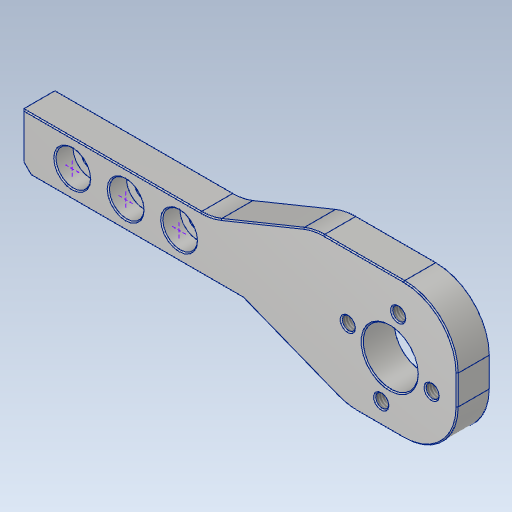
# Autodesk Inventor part: Xmovementarm
Saved by Autodesk Inventor 2020 (Build 240168000, 168)
## iProperties
Created: 2019-01-13
Part Number: Xmovementarm
Material: Aluminum 6061
Document SubType Name: Modeling
Designer: LillaHunden
Density: 2.7 g/cm^3
Appearance: Aluminum - Flat
Mass: 17.0465 g
Surface Area: 40.0048 cm^2
Volume: 6.31351 cm^3
Author: LillaHunden
Autodesk Inventor part; units mm, degrees
ref_plane "YZ Plane" through (0, 0, 0) normal (1, 0, 0) x (0, 1, 0)
ref_plane "XZ Plane" through (0, 0, 0) normal (0, 1, 0) x (-1, 0, 0)
ref_plane "XY Plane" through (0, 0, 0) normal (0, 0, 1) x (1, 0, 0)
sketch "Sketch1" plane through (0, 0, 0) normal (0, 0, 1) x (1, 0, 0)
  line L0 (86.0355, 17.7845) -> (59.096, 17.7845)
  line L1 (59.096, 17.7845) -> (59.096, 0)
  line L2 (65.4983, -7.6947) -> (86.0355, -7.6947)
  line L3 (86.0355, -7.6947) -> (86.0355, 17.7845)
  line L4 (6.25, 0) -> (40, 0) projected
  line L5 (40, 0) -> (40, 10) projected
  line L6 (4.75, 10) -> (40, 10) projected
  line L7 (40, 10) -> (59.096, 10)
  line L8 (40, 0) -> (59.096, 0)
  line L9 (59.096, 17.7845) -> (40, 10)
  circle A0 centre (34, 5) radius 2 projected
  line L10 (4.75, 10) -> (4.75, 1.5) projected
  circle A1 centre (14, 5) radius 1.5 projected
  circle A2 centre (34, 5) radius 1.5 projected
  circle A3 centre (24, 5) radius 1.5 projected
  line L11 (6.25, 0) -> (4.75, 1.5) projected
  line L12 (46, -2.9015) -> (46, 0) projected
  line L13 (65.4983, -7.6947) -> (46, 0)
  constraints: 16 end point, 3 perpendicular, 2 parallel, 1 horizontal, 1 point on line, 1 vertical alignment
extrude "Extrusion1" add sketch "Sketch1" along normal blind 6 contours L3 L2 L13 L8 L1 L0 | L1 L7 L9 | L1 L8 L5 L7 | L5 L4 L11 L10 L6 | A0 | A1 | A2 | A3
sketch "Sketch2" plane through (0, 0, 0) normal (0, 0, -1) x (-1, 0, 0)
  circle A0 centre (-73.4131, 4.0423) radius 11 construction
  spline S0 degree 3 poles (-70.2966, -4.0075) (-70.3394, -4.1944) (-70.4189, -4.3706) (-70.5284, -4.5282) (-70.5355, -4.5385) (-70.5428, -4.5487) (-70.5503, -4.5589) (-70.6442, -4.6873) (-70.7571, -4.8004) (-70.8853, -4.8928) (-70.903, -4.9055) (-70.921, -4.9179) (-70.9392, -4.9298) (-70.9477, -4.9354) (-70.9563, -4.9408) (-70.9649, -4.9462) (-71.0438, -4.9954) (-71.1272, -5.0364) (-71.2142, -5.0682) (-71.2658, -5.087) (-71.3187, -5.1025) (-71.3725, -5.1148) (-71.4037, -5.1219) (-71.4353, -5.1279) (-71.4671, -5.1328) (-71.6122, -5.1551) (-71.7606, -5.1543) (-71.906, -5.1306) (-71.9241, -5.1277) (-71.9422, -5.1244) (-71.9602, -5.1207) (-71.9711, -5.1185) (-71.9819, -5.1162) (-71.9928, -5.1137) (-72.0898, -5.0915) (-72.1841, -5.059) (-72.2734, -5.016) (-72.3457, -4.9813) (-72.4143, -4.9399) (-72.478, -4.8918) (-72.4941, -4.8797) (-72.5098, -4.8672) (-72.5244, -4.8525) knots 0 0 0 0 0.200829 0.200829 0.200829 0.213978 0.213978 0.213978 0.380655 0.380655 0.380655 0.403633 0.403633 0.403633 0.414319 0.414319 0.414319 0.512539 0.512539 0.512539 0.570815 0.570815 0.570815 0.60461 0.60461 0.60461 0.759068 0.759068 0.759068 0.77833 0.77833 0.77833 0.789949 0.789949 0.789949 0.894318 0.894318 0.894318 0.978751 0.978751 0.978751 1 1 1 1 construction
  arc A1 (-73.0648, -4.0495) -> (-72.5243, -4.8523) centre (-71.8254, -3.7985) ccw construction
  spline S1 degree 3 poles (-73.0648, -4.0495) (-73.1089, -3.9109) (-73.127, -3.7658) (-73.1216, -3.6205) (-73.121, -3.6026) (-73.12, -3.5847) (-73.1186, -3.5668) (-73.1178, -3.5567) (-73.117, -3.5466) (-73.116, -3.5366) (-73.1013, -3.3878) (-73.0625, -3.2423) (-73.0016, -3.1063) (-72.9947, -3.091) (-72.9875, -3.0757) (-72.9801, -3.0606) (-72.9752, -3.0506) (-72.9701, -3.0407) (-72.9649, -3.0308) (-72.923, -2.9506) (-72.8732, -2.8752) (-72.8161, -2.8057) (-72.7812, -2.7633) (-72.7435, -2.7231) (-72.7034, -2.6852) (-72.6914, -2.6738) (-72.6792, -2.6627) (-72.6668, -2.6518) (-72.6553, -2.6417) (-72.6436, -2.6318) (-72.6317, -2.622) (-72.5007, -2.5145) (-72.3507, -2.4308) (-72.19, -2.3729) (-72.1789, -2.3689) (-72.1678, -2.365) (-72.1566, -2.3613) (-72.062, -2.3296) (-71.9647, -2.3072) (-71.8662, -2.2944) (-71.8501, -2.2924) (-71.8341, -2.2905) (-71.818, -2.289) (-71.8062, -2.2878) (-71.7944, -2.2868) (-71.7826, -2.286) (-71.722, -2.2815) (-71.6612, -2.2808) (-71.6007, -2.2839) (-71.5723, -2.2854) (-71.544, -2.2877) (-71.5158, -2.2909) (-71.4916, -2.2936) (-71.4675, -2.297) (-71.4437, -2.3035) knots 0 0 0 0 0.153066 0.153066 0.153066 0.171917 0.171917 0.171917 0.182531 0.182531 0.182531 0.339556 0.339556 0.339556 0.35729 0.35729 0.35729 0.369023 0.369023 0.369023 0.464442 0.464442 0.464442 0.522742 0.522742 0.522742 0.540193 0.540193 0.540193 0.556325 0.556325 0.556325 0.734813 0.734813 0.734813 0.747126 0.747126 0.747126 0.851246 0.851246 0.851246 0.868176 0.868176 0.868176 0.880588 0.880588 0.880588 0.944403 0.944403 0.944403 0.974326 0.974326 0.974326 1 1 1 1 construction
  arc A2 (-70.2966, -4.0075) -> (-71.4439, -2.3035) centre (-71.8254, -3.7985) ccw construction
  spline S2 degree 3 poles (-64.0434, 5.421) (-64.0862, 5.2342) (-64.1657, 5.0579) (-64.2751, 4.9003) (-64.2823, 4.89) (-64.2896, 4.8798) (-64.297, 4.8697) (-64.404, 4.7235) (-64.5353, 4.5971) (-64.686, 4.4987) (-64.6945, 4.4932) (-64.703, 4.4877) (-64.7116, 4.4824) (-64.7906, 4.4331) (-64.874, 4.3921) (-64.9609, 4.3604) (-65.0125, 4.3415) (-65.0654, 4.326) (-65.1193, 4.3137) (-65.1359, 4.31) (-65.1526, 4.3065) (-65.1694, 4.3033) (-65.1842, 4.3006) (-65.199, 4.298) (-65.2138, 4.2957) (-65.359, 4.2734) (-65.5074, 4.2742) (-65.6528, 4.2979) (-65.6709, 4.3008) (-65.689, 4.3041) (-65.707, 4.3078) (-65.7179, 4.31) (-65.7287, 4.3124) (-65.7395, 4.3148) (-65.8246, 4.3343) (-65.9075, 4.3617) (-65.9869, 4.3971) (-65.9981, 4.402) (-66.0092, 4.4072) (-66.0202, 4.4125) (-66.0665, 4.4348) (-66.1114, 4.4598) (-66.1544, 4.4876) (-66.1784, 4.5031) (-66.2019, 4.5195) (-66.2248, 4.5367) (-66.2409, 4.5488) (-66.2566, 4.5613) (-66.2712, 4.576) knots 0 0 0 0 0.200829 0.200829 0.200829 0.213978 0.213978 0.213978 0.403633 0.403633 0.403633 0.414319 0.414319 0.414319 0.512539 0.512539 0.512539 0.570815 0.570815 0.570815 0.588808 0.588808 0.588808 0.60461 0.60461 0.60461 0.759068 0.759068 0.759068 0.77833 0.77833 0.77833 0.789949 0.789949 0.789949 0.881423 0.881423 0.881423 0.894318 0.894318 0.894318 0.948472 0.948472 0.948472 0.978751 0.978751 0.978751 1 1 1 1 construction
  arc A3 (-66.8115, 5.379) -> (-66.2711, 4.5762) centre (-65.5722, 5.63) ccw construction
  spline S3 degree 3 poles (-66.8115, 5.379) (-66.8557, 5.5177) (-66.8737, 5.6627) (-66.8684, 5.808) (-66.8678, 5.8259) (-66.8667, 5.8438) (-66.8654, 5.8617) (-66.8646, 5.8718) (-66.8637, 5.8819) (-66.8627, 5.892) (-66.848, 6.0407) (-66.8092, 6.1862) (-66.7483, 6.3222) (-66.7415, 6.3376) (-66.7343, 6.3528) (-66.7269, 6.3679) (-66.7219, 6.3779) (-66.7169, 6.3879) (-66.7117, 6.3977) (-66.6697, 6.4779) (-66.62, 6.5534) (-66.5629, 6.6228) (-66.528, 6.6653) (-66.4903, 6.7055) (-66.4502, 6.7433) (-66.4382, 6.7547) (-66.426, 6.7658) (-66.4135, 6.7767) (-66.402, 6.7868) (-66.3903, 6.7968) (-66.3785, 6.8065) (-66.2625, 6.9017) (-66.1315, 6.9782) (-65.9915, 7.0347) (-65.9734, 7.042) (-65.9552, 7.049) (-65.9368, 7.0556) (-65.8689, 7.0801) (-65.7992, 7.0998) (-65.7287, 7.1145) (-65.6904, 7.1225) (-65.6518, 7.1291) (-65.6129, 7.1341) (-65.5969, 7.1362) (-65.5809, 7.138) (-65.5648, 7.1396) (-65.553, 7.1407) (-65.5412, 7.1417) (-65.5294, 7.1426) (-65.4687, 7.147) (-65.408, 7.1477) (-65.3475, 7.1446) (-65.3191, 7.1431) (-65.2908, 7.1408) (-65.2626, 7.1376) (-65.2384, 7.1349) (-65.2142, 7.1316) (-65.1905, 7.125) knots 0 0 0 0 0.153066 0.153066 0.153066 0.171917 0.171917 0.171917 0.182531 0.182531 0.182531 0.339556 0.339556 0.339556 0.35729 0.35729 0.35729 0.369023 0.369023 0.369023 0.464442 0.464442 0.464442 0.522742 0.522742 0.522742 0.540193 0.540193 0.540193 0.556325 0.556325 0.556325 0.714368 0.714368 0.714368 0.734813 0.734813 0.734813 0.810219 0.810219 0.810219 0.851246 0.851246 0.851246 0.868176 0.868176 0.868176 0.880588 0.880588 0.880588 0.944403 0.944403 0.944403 0.974325 0.974325 0.974325 1 1 1 1 construction
  arc A4 (-64.0434, 5.421) -> (-65.1906, 7.1251) centre (-65.5722, 5.63) ccw construction
  spline S4 degree 3 poles (-73.4719, 11.6743) (-73.5094, 11.5106) (-73.5751, 11.3552) (-73.6643, 11.2132) (-73.6769, 11.193) (-73.6901, 11.1732) (-73.7037, 11.1536) (-73.7108, 11.1433) (-73.7181, 11.133) (-73.7255, 11.1229) (-73.8195, 10.9944) (-73.9324, 10.8814) (-74.0606, 10.789) (-74.0783, 10.7762) (-74.0963, 10.7639) (-74.1145, 10.752) (-74.123, 10.7464) (-74.1315, 10.741) (-74.1401, 10.7356) (-74.2191, 10.6864) (-74.3025, 10.6453) (-74.3895, 10.6136) (-74.4411, 10.5948) (-74.4939, 10.5792) (-74.5478, 10.567) (-74.5644, 10.5632) (-74.5811, 10.5597) (-74.5979, 10.5566) (-74.7569, 10.5267) (-74.921, 10.5251) (-75.0813, 10.5511) (-75.0994, 10.5541) (-75.1175, 10.5574) (-75.1355, 10.561) (-75.1464, 10.5633) (-75.1572, 10.5656) (-75.168, 10.5681) (-75.2531, 10.5875) (-75.3361, 10.6149) (-75.4154, 10.6503) (-75.4266, 10.6553) (-75.4377, 10.6604) (-75.4487, 10.6657) (-75.521, 10.7005) (-75.5896, 10.7418) (-75.6533, 10.7899) (-75.6694, 10.802) (-75.6851, 10.8146) (-75.6997, 10.8292) knots 0 0 0 0 0.175859 0.175859 0.175859 0.200829 0.200829 0.200829 0.213978 0.213978 0.213978 0.380655 0.380655 0.380655 0.403633 0.403633 0.403633 0.414319 0.414319 0.414319 0.512539 0.512539 0.512539 0.570815 0.570815 0.570815 0.588808 0.588808 0.588808 0.759068 0.759068 0.759068 0.77833 0.77833 0.77833 0.789949 0.789949 0.789949 0.881423 0.881423 0.881423 0.894318 0.894318 0.894318 0.978751 0.978751 0.978751 1 1 1 1 construction
  arc A5 (-76.2401, 11.6323) -> (-75.6996, 10.8294) centre (-75.0007, 11.8832) ccw construction
  spline S5 degree 3 poles (-76.2401, 11.6323) (-76.2927, 11.7976) (-76.3084, 11.9722) (-76.2913, 12.1452) (-76.2765, 12.294) (-76.2378, 12.4394) (-76.1769, 12.5754) (-76.17, 12.5908) (-76.1628, 12.606) (-76.1554, 12.6212) (-76.1505, 12.6312) (-76.1454, 12.6411) (-76.1402, 12.6509) (-76.0982, 12.7311) (-76.0485, 12.8066) (-75.9914, 12.8761) (-75.9565, 12.9185) (-75.9188, 12.9587) (-75.8787, 12.9966) (-75.8667, 13.0079) (-75.8545, 13.019) (-75.842, 13.03) (-75.8305, 13.0401) (-75.8189, 13.05) (-75.807, 13.0597) (-75.691, 13.155) (-75.5601, 13.2315) (-75.4201, 13.288) (-75.402, 13.2953) (-75.3837, 13.3022) (-75.3653, 13.3089) (-75.3542, 13.3129) (-75.3431, 13.3167) (-75.3319, 13.3205) (-75.2373, 13.3521) (-75.14, 13.3746) (-75.0415, 13.3873) (-75.0254, 13.3894) (-75.0094, 13.3912) (-74.9933, 13.3928) (-74.9815, 13.3939) (-74.9697, 13.3949) (-74.9579, 13.3958) (-74.8688, 13.4023) (-74.7795, 13.4008) (-74.6911, 13.3909) (-74.6669, 13.3882) (-74.6427, 13.3848) (-74.619, 13.3783) knots 0 0 0 0 0.182531 0.182531 0.182531 0.339556 0.339556 0.339556 0.357289 0.357289 0.357289 0.369023 0.369023 0.369023 0.464442 0.464442 0.464442 0.522742 0.522742 0.522742 0.540193 0.540193 0.540193 0.556325 0.556325 0.556325 0.714368 0.714368 0.714368 0.734813 0.734813 0.734813 0.747125 0.747125 0.747125 0.851246 0.851246 0.851246 0.868176 0.868176 0.868176 0.880588 0.880588 0.880588 0.974325 0.974325 0.974325 1 1 1 1 construction
  arc A6 (-73.4719, 11.6743) -> (-74.6192, 13.3783) centre (-75.0007, 11.8832) ccw construction
  spline S6 degree 3 poles (-79.7252, 2.2457) (-79.8062, 1.8916) (-80.0211, 1.5714) (-80.3139, 1.3604) (-80.3315, 1.3477) (-80.3495, 1.3354) (-80.3677, 1.3234) (-80.3762, 1.3179) (-80.3848, 1.3124) (-80.3934, 1.3071) (-80.4724, 1.2579) (-80.5557, 1.2168) (-80.6427, 1.1851) (-80.6943, 1.1662) (-80.7472, 1.1507) (-80.801, 1.1385) (-80.8177, 1.1347) (-80.8344, 1.1312) (-80.8512, 1.128) (-80.8659, 1.1253) (-80.8807, 1.1227) (-80.8956, 1.1204) (-81.0408, 1.0981) (-81.1891, 1.0989) (-81.3345, 1.1226) (-81.3526, 1.1256) (-81.3707, 1.1289) (-81.3888, 1.1325) (-81.3996, 1.1347) (-81.4105, 1.1371) (-81.4213, 1.1395) (-81.5064, 1.159) (-81.5893, 1.1864) (-81.6686, 1.2218) (-81.6798, 1.2268) (-81.6909, 1.2319) (-81.702, 1.2372) (-81.7742, 1.2719) (-81.8428, 1.3133) (-81.9066, 1.3614) (-81.9226, 1.3735) (-81.9384, 1.3861) (-81.953, 1.4007) knots 0 0 0 0 0.380655 0.380655 0.380655 0.403633 0.403633 0.403633 0.414319 0.414319 0.414319 0.512539 0.512539 0.512539 0.570815 0.570815 0.570815 0.588808 0.588808 0.588808 0.60461 0.60461 0.60461 0.759068 0.759068 0.759068 0.77833 0.77833 0.77833 0.789949 0.789949 0.789949 0.881423 0.881423 0.881423 0.894318 0.894318 0.894318 0.978751 0.978751 0.978751 1 1 1 1 construction
  arc A7 (-82.4933, 2.2038) -> (-81.9529, 1.4009) centre (-81.2539, 2.4547) ccw construction
  spline S7 degree 3 poles (-82.4933, 2.2038) (-82.5374, 2.3424) (-82.5555, 2.4874) (-82.5502, 2.6328) (-82.5495, 2.6507) (-82.5485, 2.6686) (-82.5471, 2.6865) (-82.5464, 2.6965) (-82.5455, 2.7066) (-82.5445, 2.7167) (-82.5281, 2.8823) (-82.482, 3.0437) (-82.4086, 3.1926) (-82.4037, 3.2026) (-82.3986, 3.2126) (-82.3935, 3.2224) (-82.3515, 3.3026) (-82.3017, 3.3781) (-82.2446, 3.4475) (-82.2097, 3.49) (-82.1721, 3.5302) (-82.132, 3.5681) (-82.1199, 3.5794) (-82.1077, 3.5905) (-82.0953, 3.6014) (-82.0838, 3.6115) (-82.0721, 3.6215) (-82.0603, 3.6312) (-81.9292, 3.7388) (-81.7792, 3.8225) (-81.6185, 3.8803) (-81.6074, 3.8843) (-81.5963, 3.8882) (-81.5851, 3.892) (-81.4752, 3.9287) (-81.3615, 3.9531) (-81.2465, 3.9643) (-81.2348, 3.9654) (-81.223, 3.9664) (-81.2111, 3.9673) (-81.1505, 3.9717) (-81.0897, 3.9724) (-81.0292, 3.9693) (-81.0009, 3.9678) (-80.9726, 3.9655) (-80.9443, 3.9624) (-80.9201, 3.9596) (-80.896, 3.9563) (-80.8722, 3.9497) knots 0 0 0 0 0.153066 0.153066 0.153066 0.171917 0.171917 0.171917 0.182531 0.182531 0.182531 0.357289 0.357289 0.357289 0.369023 0.369023 0.369023 0.464442 0.464442 0.464442 0.522742 0.522742 0.522742 0.540193 0.540193 0.540193 0.556325 0.556325 0.556325 0.734813 0.734813 0.734813 0.747125 0.747125 0.747125 0.868176 0.868176 0.868176 0.880588 0.880588 0.880588 0.944403 0.944403 0.944403 0.974325 0.974325 0.974325 1 1 1 1 construction
  arc A8 (-79.7252, 2.2457) -> (-80.8724, 3.9498) centre (-81.2539, 2.4547) ccw construction
  circle A9 centre (-73.4131, 4.0423) radius 5.15 construction
  point P0 (0, 0)
  constraints: 4 coincident
hole "Hole1" at (81.2539, 2.4547, 0) at (75.0007, 11.8832, 0) at (65.5722, 5.63, 0) at (71.8254, -3.7985, 0) direction (0, 0, 1) diameter 2.459 depth 8.8 thread size "M3x0.5" class "6H" standard "ISO Metric profile"
sketch "Sketch3" plane through (0, 0, 6) normal (0, 0, 1) x (1, 0, 0)
  circle A0 centre (73.4131, 4.0423) radius 11
  spline S0 degree 3 poles (70.2966, -4.0075) (70.3394, -4.1944) (70.4189, -4.3706) (70.5284, -4.5282) (70.5355, -4.5385) (70.5428, -4.5487) (70.5503, -4.5589) (70.6442, -4.6873) (70.7571, -4.8004) (70.8853, -4.8928) (70.903, -4.9055) (70.921, -4.9179) (70.9392, -4.9298) (70.9477, -4.9354) (70.9563, -4.9408) (70.9649, -4.9462) (71.0438, -4.9954) (71.1272, -5.0364) (71.2142, -5.0682) (71.2658, -5.087) (71.3187, -5.1025) (71.3725, -5.1148) (71.4037, -5.1219) (71.4353, -5.1279) (71.4671, -5.1328) (71.6122, -5.1551) (71.7606, -5.1543) (71.906, -5.1306) (71.9241, -5.1277) (71.9422, -5.1244) (71.9602, -5.1207) (71.9711, -5.1185) (71.9819, -5.1162) (71.9928, -5.1137) (72.0898, -5.0915) (72.1841, -5.059) (72.2734, -5.016) (72.3457, -4.9813) (72.4143, -4.9399) (72.478, -4.8918) (72.4941, -4.8797) (72.5098, -4.8672) (72.5244, -4.8525) knots 0 0 0 0 0.200829 0.200829 0.200829 0.213978 0.213978 0.213978 0.380655 0.380655 0.380655 0.403633 0.403633 0.403633 0.414319 0.414319 0.414319 0.512539 0.512539 0.512539 0.570815 0.570815 0.570815 0.60461 0.60461 0.60461 0.759068 0.759068 0.759068 0.77833 0.77833 0.77833 0.789949 0.789949 0.789949 0.894318 0.894318 0.894318 0.978751 0.978751 0.978751 1 1 1 1
  arc A1 (72.5243, -4.8523) -> (73.0648, -4.0495) centre (71.8254, -3.7985) ccw
  spline S1 degree 3 poles (73.0648, -4.0495) (73.1089, -3.9109) (73.127, -3.7658) (73.1216, -3.6205) (73.121, -3.6026) (73.12, -3.5847) (73.1186, -3.5668) (73.1178, -3.5567) (73.117, -3.5466) (73.116, -3.5366) (73.1013, -3.3878) (73.0625, -3.2423) (73.0016, -3.1063) (72.9947, -3.091) (72.9875, -3.0757) (72.9801, -3.0606) (72.9752, -3.0506) (72.9701, -3.0407) (72.9649, -3.0308) (72.923, -2.9506) (72.8732, -2.8752) (72.8161, -2.8057) (72.7812, -2.7633) (72.7435, -2.7231) (72.7034, -2.6852) (72.6914, -2.6738) (72.6792, -2.6627) (72.6668, -2.6518) (72.6553, -2.6417) (72.6436, -2.6318) (72.6317, -2.622) (72.5007, -2.5145) (72.3507, -2.4308) (72.19, -2.3729) (72.1789, -2.3689) (72.1678, -2.365) (72.1566, -2.3613) (72.062, -2.3296) (71.9647, -2.3072) (71.8662, -2.2944) (71.8501, -2.2924) (71.8341, -2.2905) (71.818, -2.289) (71.8062, -2.2878) (71.7944, -2.2868) (71.7826, -2.286) (71.722, -2.2815) (71.6612, -2.2808) (71.6007, -2.2839) (71.5723, -2.2854) (71.544, -2.2877) (71.5158, -2.2909) (71.4916, -2.2936) (71.4675, -2.297) (71.4437, -2.3035) knots 0 0 0 0 0.153066 0.153066 0.153066 0.171917 0.171917 0.171917 0.182531 0.182531 0.182531 0.339556 0.339556 0.339556 0.35729 0.35729 0.35729 0.369023 0.369023 0.369023 0.464442 0.464442 0.464442 0.522742 0.522742 0.522742 0.540193 0.540193 0.540193 0.556325 0.556325 0.556325 0.734813 0.734813 0.734813 0.747126 0.747126 0.747126 0.851246 0.851246 0.851246 0.868176 0.868176 0.868176 0.880588 0.880588 0.880588 0.944403 0.944403 0.944403 0.974326 0.974326 0.974326 1 1 1 1
  arc A2 (71.4439, -2.3035) -> (70.2966, -4.0075) centre (71.8254, -3.7985) ccw
  spline S2 degree 3 poles (64.0434, 5.421) (64.0862, 5.2342) (64.1657, 5.0579) (64.2751, 4.9003) (64.2823, 4.89) (64.2896, 4.8798) (64.297, 4.8697) (64.404, 4.7235) (64.5353, 4.5971) (64.686, 4.4987) (64.6945, 4.4932) (64.703, 4.4877) (64.7116, 4.4824) (64.7906, 4.4331) (64.874, 4.3921) (64.9609, 4.3604) (65.0125, 4.3415) (65.0654, 4.326) (65.1193, 4.3137) (65.1359, 4.31) (65.1526, 4.3065) (65.1694, 4.3033) (65.1842, 4.3006) (65.199, 4.298) (65.2138, 4.2957) (65.359, 4.2734) (65.5074, 4.2742) (65.6528, 4.2979) (65.6709, 4.3008) (65.689, 4.3041) (65.707, 4.3078) (65.7179, 4.31) (65.7287, 4.3124) (65.7395, 4.3148) (65.8246, 4.3343) (65.9075, 4.3617) (65.9869, 4.3971) (65.9981, 4.402) (66.0092, 4.4072) (66.0202, 4.4125) (66.0665, 4.4348) (66.1114, 4.4598) (66.1544, 4.4876) (66.1784, 4.5031) (66.2019, 4.5195) (66.2248, 4.5367) (66.2409, 4.5488) (66.2566, 4.5613) (66.2712, 4.576) knots 0 0 0 0 0.200829 0.200829 0.200829 0.213978 0.213978 0.213978 0.403633 0.403633 0.403633 0.414319 0.414319 0.414319 0.512539 0.512539 0.512539 0.570815 0.570815 0.570815 0.588808 0.588808 0.588808 0.60461 0.60461 0.60461 0.759068 0.759068 0.759068 0.77833 0.77833 0.77833 0.789949 0.789949 0.789949 0.881423 0.881423 0.881423 0.894318 0.894318 0.894318 0.948472 0.948472 0.948472 0.978751 0.978751 0.978751 1 1 1 1
  arc A3 (66.2711, 4.5762) -> (66.8115, 5.379) centre (65.5722, 5.63) ccw
  spline S3 degree 3 poles (66.8115, 5.379) (66.8557, 5.5177) (66.8737, 5.6627) (66.8684, 5.808) (66.8678, 5.8259) (66.8667, 5.8438) (66.8654, 5.8617) (66.8646, 5.8718) (66.8637, 5.8819) (66.8627, 5.892) (66.848, 6.0407) (66.8092, 6.1862) (66.7483, 6.3222) (66.7415, 6.3376) (66.7343, 6.3528) (66.7269, 6.3679) (66.7219, 6.3779) (66.7169, 6.3879) (66.7117, 6.3977) (66.6697, 6.4779) (66.62, 6.5534) (66.5629, 6.6228) (66.528, 6.6653) (66.4903, 6.7055) (66.4502, 6.7433) (66.4382, 6.7547) (66.426, 6.7658) (66.4135, 6.7767) (66.402, 6.7868) (66.3903, 6.7968) (66.3785, 6.8065) (66.2625, 6.9017) (66.1315, 6.9782) (65.9915, 7.0347) (65.9734, 7.042) (65.9552, 7.049) (65.9368, 7.0556) (65.8689, 7.0801) (65.7992, 7.0998) (65.7287, 7.1145) (65.6904, 7.1225) (65.6518, 7.1291) (65.6129, 7.1341) (65.5969, 7.1362) (65.5809, 7.138) (65.5648, 7.1396) (65.553, 7.1407) (65.5412, 7.1417) (65.5294, 7.1426) (65.4687, 7.147) (65.408, 7.1477) (65.3475, 7.1446) (65.3191, 7.1431) (65.2908, 7.1408) (65.2626, 7.1376) (65.2384, 7.1349) (65.2142, 7.1316) (65.1905, 7.125) knots 0 0 0 0 0.153066 0.153066 0.153066 0.171917 0.171917 0.171917 0.182531 0.182531 0.182531 0.339556 0.339556 0.339556 0.35729 0.35729 0.35729 0.369023 0.369023 0.369023 0.464442 0.464442 0.464442 0.522742 0.522742 0.522742 0.540193 0.540193 0.540193 0.556325 0.556325 0.556325 0.714368 0.714368 0.714368 0.734813 0.734813 0.734813 0.810219 0.810219 0.810219 0.851246 0.851246 0.851246 0.868176 0.868176 0.868176 0.880588 0.880588 0.880588 0.944403 0.944403 0.944403 0.974325 0.974325 0.974325 1 1 1 1
  arc A4 (65.1906, 7.1251) -> (64.0434, 5.421) centre (65.5722, 5.63) ccw
  spline S4 degree 3 poles (73.4719, 11.6743) (73.5094, 11.5106) (73.5751, 11.3552) (73.6643, 11.2132) (73.6769, 11.193) (73.6901, 11.1732) (73.7037, 11.1536) (73.7108, 11.1433) (73.7181, 11.133) (73.7255, 11.1229) (73.8195, 10.9944) (73.9324, 10.8814) (74.0606, 10.789) (74.0783, 10.7762) (74.0963, 10.7639) (74.1145, 10.752) (74.123, 10.7464) (74.1315, 10.741) (74.1401, 10.7356) (74.2191, 10.6864) (74.3025, 10.6453) (74.3895, 10.6136) (74.4411, 10.5948) (74.4939, 10.5792) (74.5478, 10.567) (74.5644, 10.5632) (74.5811, 10.5597) (74.5979, 10.5566) (74.7569, 10.5267) (74.921, 10.5251) (75.0813, 10.5511) (75.0994, 10.5541) (75.1175, 10.5574) (75.1355, 10.561) (75.1464, 10.5633) (75.1572, 10.5656) (75.168, 10.5681) (75.2531, 10.5875) (75.3361, 10.6149) (75.4154, 10.6503) (75.4266, 10.6553) (75.4377, 10.6604) (75.4487, 10.6657) (75.521, 10.7005) (75.5896, 10.7418) (75.6533, 10.7899) (75.6694, 10.802) (75.6851, 10.8146) (75.6997, 10.8292) knots 0 0 0 0 0.175859 0.175859 0.175859 0.200829 0.200829 0.200829 0.213978 0.213978 0.213978 0.380655 0.380655 0.380655 0.403633 0.403633 0.403633 0.414319 0.414319 0.414319 0.512539 0.512539 0.512539 0.570815 0.570815 0.570815 0.588808 0.588808 0.588808 0.759068 0.759068 0.759068 0.77833 0.77833 0.77833 0.789949 0.789949 0.789949 0.881423 0.881423 0.881423 0.894318 0.894318 0.894318 0.978751 0.978751 0.978751 1 1 1 1
  arc A5 (75.6996, 10.8294) -> (76.2401, 11.6323) centre (75.0007, 11.8832) ccw
  spline S5 degree 3 poles (76.2401, 11.6323) (76.2927, 11.7976) (76.3084, 11.9722) (76.2913, 12.1452) (76.2765, 12.294) (76.2378, 12.4394) (76.1769, 12.5754) (76.17, 12.5908) (76.1628, 12.606) (76.1554, 12.6212) (76.1505, 12.6312) (76.1454, 12.6411) (76.1402, 12.6509) (76.0982, 12.7311) (76.0485, 12.8066) (75.9914, 12.8761) (75.9565, 12.9185) (75.9188, 12.9587) (75.8787, 12.9966) (75.8667, 13.0079) (75.8545, 13.019) (75.842, 13.03) (75.8305, 13.0401) (75.8189, 13.05) (75.807, 13.0597) (75.691, 13.155) (75.5601, 13.2315) (75.4201, 13.288) (75.402, 13.2953) (75.3837, 13.3022) (75.3653, 13.3089) (75.3542, 13.3129) (75.3431, 13.3167) (75.3319, 13.3205) (75.2373, 13.3521) (75.14, 13.3746) (75.0415, 13.3873) (75.0254, 13.3894) (75.0094, 13.3912) (74.9933, 13.3928) (74.9815, 13.3939) (74.9697, 13.3949) (74.9579, 13.3958) (74.8688, 13.4023) (74.7795, 13.4008) (74.6911, 13.3909) (74.6669, 13.3882) (74.6427, 13.3848) (74.619, 13.3783) knots 0 0 0 0 0.182531 0.182531 0.182531 0.339556 0.339556 0.339556 0.357289 0.357289 0.357289 0.369023 0.369023 0.369023 0.464442 0.464442 0.464442 0.522742 0.522742 0.522742 0.540193 0.540193 0.540193 0.556325 0.556325 0.556325 0.714368 0.714368 0.714368 0.734813 0.734813 0.734813 0.747125 0.747125 0.747125 0.851246 0.851246 0.851246 0.868176 0.868176 0.868176 0.880588 0.880588 0.880588 0.974325 0.974325 0.974325 1 1 1 1
  arc A6 (74.6192, 13.3783) -> (73.4719, 11.6743) centre (75.0007, 11.8832) ccw
  spline S6 degree 3 poles (79.7252, 2.2457) (79.8062, 1.8916) (80.0211, 1.5714) (80.3139, 1.3604) (80.3315, 1.3477) (80.3495, 1.3354) (80.3677, 1.3234) (80.3762, 1.3179) (80.3848, 1.3124) (80.3934, 1.3071) (80.4724, 1.2579) (80.5557, 1.2168) (80.6427, 1.1851) (80.6943, 1.1662) (80.7472, 1.1507) (80.801, 1.1385) (80.8177, 1.1347) (80.8344, 1.1312) (80.8512, 1.128) (80.8659, 1.1253) (80.8807, 1.1227) (80.8956, 1.1204) (81.0408, 1.0981) (81.1891, 1.0989) (81.3345, 1.1226) (81.3526, 1.1256) (81.3707, 1.1289) (81.3888, 1.1325) (81.3996, 1.1347) (81.4105, 1.1371) (81.4213, 1.1395) (81.5064, 1.159) (81.5893, 1.1864) (81.6686, 1.2218) (81.6798, 1.2268) (81.6909, 1.2319) (81.702, 1.2372) (81.7742, 1.2719) (81.8428, 1.3133) (81.9066, 1.3614) (81.9226, 1.3735) (81.9384, 1.3861) (81.953, 1.4007) knots 0 0 0 0 0.380655 0.380655 0.380655 0.403633 0.403633 0.403633 0.414319 0.414319 0.414319 0.512539 0.512539 0.512539 0.570815 0.570815 0.570815 0.588808 0.588808 0.588808 0.60461 0.60461 0.60461 0.759068 0.759068 0.759068 0.77833 0.77833 0.77833 0.789949 0.789949 0.789949 0.881423 0.881423 0.881423 0.894318 0.894318 0.894318 0.978751 0.978751 0.978751 1 1 1 1
  arc A7 (81.9529, 1.4009) -> (82.4933, 2.2038) centre (81.2539, 2.4547) ccw
  spline S7 degree 3 poles (82.4933, 2.2038) (82.5374, 2.3424) (82.5555, 2.4874) (82.5502, 2.6328) (82.5495, 2.6507) (82.5485, 2.6686) (82.5471, 2.6865) (82.5464, 2.6965) (82.5455, 2.7066) (82.5445, 2.7167) (82.5281, 2.8823) (82.482, 3.0437) (82.4086, 3.1926) (82.4037, 3.2026) (82.3986, 3.2126) (82.3935, 3.2224) (82.3515, 3.3026) (82.3017, 3.3781) (82.2446, 3.4475) (82.2097, 3.49) (82.1721, 3.5302) (82.132, 3.5681) (82.1199, 3.5794) (82.1077, 3.5905) (82.0953, 3.6014) (82.0838, 3.6115) (82.0721, 3.6215) (82.0603, 3.6312) (81.9292, 3.7388) (81.7792, 3.8225) (81.6185, 3.8803) (81.6074, 3.8843) (81.5963, 3.8882) (81.5851, 3.892) (81.4752, 3.9287) (81.3615, 3.9531) (81.2465, 3.9643) (81.2348, 3.9654) (81.223, 3.9664) (81.2111, 3.9673) (81.1505, 3.9717) (81.0897, 3.9724) (81.0292, 3.9693) (81.0009, 3.9678) (80.9726, 3.9655) (80.9443, 3.9624) (80.9201, 3.9596) (80.896, 3.9563) (80.8722, 3.9497) knots 0 0 0 0 0.153066 0.153066 0.153066 0.171917 0.171917 0.171917 0.182531 0.182531 0.182531 0.357289 0.357289 0.357289 0.369023 0.369023 0.369023 0.464442 0.464442 0.464442 0.522742 0.522742 0.522742 0.540193 0.540193 0.540193 0.556325 0.556325 0.556325 0.734813 0.734813 0.734813 0.747125 0.747125 0.747125 0.868176 0.868176 0.868176 0.880588 0.880588 0.880588 0.944403 0.944403 0.944403 0.974325 0.974325 0.974325 1 1 1 1
  arc A8 (80.8724, 3.9498) -> (79.7252, 2.2457) centre (81.2539, 2.4547) ccw
  circle A9 centre (73.4131, 4.0423) radius 5.15
  point P0 (0, 0)
extrude "Extrusion2" cut sketch "Sketch3" against normal through all contours A9
sketch "Sketch4" plane through (0, 0, 6) normal (0, 0, 1) x (1, 0, 0)
  line L0 (4.75, 10) -> (4.75, 1.5) projected
  line L1 (4.75, 5.75) -> (48.7838, 5.75) construction
  point P0 (4.75, 0)
  point P1 (14.75, 5.75)
  point P2 (24.75, 5.75)
  point P3 (34.75, 5.75)
  dimension "d38" = 10
  dimension "d39" = 10
  dimension "d40" = 10
  constraints: 3 point on line, 2 end point, 1 horizontal, 1 midpoint
  measures "d38" distance of point (14.75, 5.75) L1.start
  measures "d39" distance of point (24.75, 5.75) point (14.75, 5.75)
  measures "d40" distance of point (34.75, 5.75) point (24.75, 5.75)
sketch "Sketch7" plane through (0, 0, 6) normal (0, 0, 1) x (1, 0, 0)
  point P0 (14, 5)
  point P1 (24, 5)
  point P2 (34, 5)
sketch "Sketch8" plane through (0, 0, 6) normal (0, 0, 1) x (1, 0, 0)
  point P0 (34, 5)
  point P1 (14, 5)
  point P2 (24, 5)
hole "Hole5" at (34, 5, 6) at (14, 5, 6) at (24, 5, 6) direction (0, 0, -1) diameter 3.4 depth 6 counterbore diameter 6.5 counterbore depth 3.4
fillet "Fillet1" radius 10 3 edges at (40, 10, 3) (65.4983, -7.6947, 3) (59.096, 17.7845, 3)
fillet "Fillet2" radius 10 2 edges at (86.0355, -7.6947, 3) (86.0355, 17.7845, 3)
chamfer "Chamfer1" distance 0.2 angle 45 22 edges at (54.8646, -3.4983, 6) (65.5318, -7.5186, 6) (71.7178, -7.6947, 6) (83.1065, -4.7657, 6) (86.0355, 5.0449, 6) (83.1065, 14.8556, 6) (68.5457, 17.7845, 6) (59.1326, 17.5978, 6) (49.548, 13.8922, 6) (39.9634, 10.1867, 6) (21.395, 10, 6) (26.125, 0, 6) (4.75, 5.75, 6) (5.5, 0.75, 6) (68.2631, 4.0423, 6) (71.8254, -5.028, 6) (65.5722, 4.4005, 6) (75.0007, 10.6537, 6) (81.2539, 1.2252, 6) (34, 8.25, 6) (24, 8.25, 6) (14, 8.25, 6)
equation "\"d13\" = d11"
equation "\"d11\" = 14"
body "Solid1"
